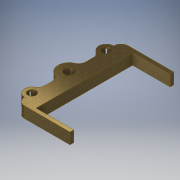
# Autodesk Inventor part: AlteredPlatformATEdit
Saved by Autodesk Inventor 2018 (Build 220112000, 112)
## iProperties
Created: 2017-10-12
Part Number: AlteredPlatformATEdit
Material: Generic
Document SubType Name: Modeling
Designer: 1452927
Density: 1 g/cm^3
Appearance: Foil Gold
Author: 1452927
Autodesk Inventor part; units mm, degrees
ref_plane "YZ Plane" through (0, 0, 0) normal (1, 0, 0) x (0, 1, 0)
sketch "Sketch1" plane through (0, 0, 0) normal (0, 1, 0) x (-1, 0, 0)
  circle A0 centre (0, 0) radius 8.0645
  circle A1 centre (0, -63.5) radius 6.985
  circle A2 centre (0, 63.5) radius 6.985
  line L0 (-39.6048, 88.9) -> (39.6048, 88.9)
  line L1 (39.6048, 88.9) -> (39.6048, -88.9)
  line L2 (39.6048, -88.9) -> (-39.6048, -88.9)
  line L3 (-39.6048, -88.9) -> (-39.6048, 88.9)
  line L4 (-39.6048, 88.9) -> (39.6048, -88.9) construction
  line L5 (39.6048, 88.9) -> (-39.6048, -88.9) construction
  line L6 (10.9754, 63.5) -> (10.9754, 0) construction
  point P0 (0, 0)
  point P1 (0, 0)
  point P2 (0, 63.5)
  dimension "d0" = 16.129
  dimension "d1" = 13.97
  dimension "d2" = 13.97
  dimension "d28" = 177.8
  dimension "d30" = 25.4
  dimension "d31" = 25.4
  constraints: 14 end point, 4 midpoint, 3 centre point, 2 coincident, 2 parallel, 1 horizontal, 1 perpendicular, 1 vertical, 4 other
  measures "d0" diameter of A0
  measures "d1" diameter of A1
  measures "d2" diameter of A2
  measures "d28" distance of L0.end L1.end
  measures "d30" distance from line of L0 point (0, 63.5)
  measures "d31" distance from line of L2 point (0, -63.5)
extrude "Extrusion4" add sketch "Sketch1" along normal blind 19.05
ref_plane "Work Plane2" through (0, 19.05, 0) normal (0, 1, 0) x (1, 0, 0)
sketch "Sketch2" plane through (0, 19.05, 0) normal (0, 1, 0) x (1, 0, 0)
  circle A0 centre (-11.2395, 0) radius 1.25
  circle A1 centre (0, 0) radius 7.94 projected
  circle A2 centre (5.6197, -9.7337) radius 1.25
  circle A3 centre (5.6198, 9.7337) radius 1.25
  dimension "d11" = 2.5
  dimension "d12" = 11.2395
  dimension "d15" = 360
  constraints: 3 centre point, 7 other
  measures "d11" diameter of A0
  measures "d12" distance of A0.centre A1.centre
ref_plane "Work Plane1" through (0, 19.05, 0) normal (0, 1, 0) x (1, 0, 0)
extrude "Extrusion5" cut sketch "Sketch2" against normal up to next contours A0 | A2 | A3
sketch "Sketch6" plane through (0, 19.05, 0) normal (0, 1, 0) x (1, 0, 0)
  line L0 (0, -38.1) -> (0, -18.8395)
  line L1 (0, 18.8395) -> (0, 38.1)
  line L2 (39.6048, 88.9) -> (-39.6048, 88.9) projected
  line L3 (0, 88.9) -> (-39.6048, 88.9)
  line L4 (-39.6048, -88.9) -> (39.6048, -88.9) projected
  line L5 (-39.6048, 88.9) -> (-39.6048, -88.9)
  line L6 (-39.6048, -88.9) -> (0, -88.9)
  circle A0 centre (0, 0) radius 8.0645 projected
  arc A1 (0, 18.8395) -> (0, -18.8395) centre (0, 0) ccw
  arc A2 (0, -50.8) -> (0, -76.2) centre (0, -63.5) ccw
  line L7 (0, -38.1) -> (0, -50.8)
  line L8 (0, -76.2) -> (0, -88.9)
  arc A3 (0, 76.2) -> (0, 50.8) centre (0, 63.5) ccw
  line L9 (0, 88.9) -> (0, 76.2)
  line L10 (0, 50.8) -> (0, 38.1)
  circle A4 centre (0, 63.5) radius 6.477
  circle A5 centre (0, -63.5) radius 6.477
  circle A6 centre (-11.2395, 0) radius 1.25 projected
  point P0 (0, 0)
  dimension "d41" = 25.4
  dimension "d42" = 25.4
  dimension "d44" = 12.954
  dimension "d45" = 12.954
  dimension "d77" = 6.35
  constraints: 18 end point, 6 point on circle, 5 centre point, 4 coincident, 4 point on line, 3 collinear, 3 vertical, 2 midpoint, 1 perpendicular
  measures "d41" diameter of A2
  measures "d42" diameter of A3
  measures "d44" diameter of A4
  measures "d45" diameter of A5
extrude "Extrusion6" cut sketch "Sketch6" against normal blind 19.05 contours L7 A2 L8 L4 L5 L2 L9 A3 L10 L1 A1 L0
fillet "Fillet5" radius 12.7 4 edges at (0, 9.525, 50.8) (0, 9.525, -50.8) (0, 9.525, -18.8395) (0, 9.525, 18.8395)
sketch "Sketch8" plane through (0, 19.05, -88.9) normal (-1, 0, 0) x (0, 0, 1)
  line L0 (33.355, -16.3528) -> (33.355, -2.5052) projected
  line L1 (15.575, -2.511) -> (15.575, -16.351) projected
  line L2 (27.5747, -16.3528) -> (27.5747, -2.5052)
  line L3 (21.1759, -16.351) -> (21.1759, -2.511)
  line L4 (33.355, -16.3528) -> (27.5747, -16.3528)
  line L5 (33.355, -2.5052) -> (27.5747, -2.5052)
  line L6 (15.575, -16.351) -> (21.1759, -16.351)
  line L7 (21.1759, -2.511) -> (15.575, -2.511)
  point P0 (88.9, -19.05)
  constraints: 12 end point, 2 parallel, 1 horizontal, 1 perpendicular
extrude "Extrusion7" cut sketch "Sketch8" along normal up to next
mirror "Mirror1" about plane through (0, 0, 0) normal (0, 0, 1) of "Extrusion7"
fillet "Fillet6" radius 12.7 2 edges at (0, 9.525, 88.9) (0, 9.525, -88.9)
sketch "Sketch12" plane through (0, 19.05, 0) normal (0, 1, 0) x (1, 0, 0)
  line L0 (39.6048, -88.9) -> (39.6048, 88.9) projected
  line L1 (39.6048, -82.55) -> (19.685, -82.55)
  line L2 (19.685, -82.55) -> (19.685, 82.55)
  line L3 (19.685, 82.55) -> (39.6048, 82.55)
  line L4 (39.6048, 82.55) -> (39.6048, -82.55)
  line L5 (39.6048, 88.9) -> (12.7, 88.9) projected
  line L6 (12.7, -88.9) -> (39.6048, -88.9) projected
  circle A0 centre (0, -63.5) radius 6.985 projected
  point P0 (0, 0)
  dimension "d72" = 6.35
  dimension "d73" = 6.35
  dimension "d74" = 12.7
  constraints: 8 end point, 2 parallel, 1 horizontal, 1 perpendicular, 1 point on line
  measures "d72" distance between parallel lines of L5 L3
  measures "d73" distance between parallel lines of L1 L6
  measures "d74" distance edge to line of A0 L2
extrude "Extrusion10" cut sketch "Sketch12" against normal up to next contours L1 L2 L3 L0
sketch "Sketch13" plane through (39.6048, 0, 88.9) normal (1, 0, 0) x (0, 0, -1)
  line L0 (0, 0) -> (0, 19.05) projected
  line L1 (171.45, 0) -> (6.35, 0) projected
  line L2 (0, 19.05) -> (6.35, 19.05)
  line L3 (6.35, 19.05) -> (6.35, 0)
  line L4 (6.35, 0) -> (0, 0)
  line L5 (0, 0) -> (0, 19.05)
  line L6 (171.45, 19.05) -> (171.45, 0) projected
  line L7 (177.8, 19.05) -> (177.8, 0) projected
  line L8 (171.45, 19.05) -> (177.8, 19.05)
  line L9 (177.8, 19.05) -> (177.8, 0)
  line L10 (177.8, 0) -> (171.45, 0)
  line L11 (171.45, 0) -> (171.45, 19.05)
  point P0 (88.9, 0)
  constraints: 16 end point, 4 parallel, 2 horizontal, 2 perpendicular
extrude "Extrusion11" add sketch "Sketch13" along normal blind 50.8
sketch "Sketch14" plane through (19.685, 19.05, 82.55) normal (1, 0, 0) x (0, 0, -1)
  line L0 (0, -19.05) -> (0, 0) projected
  line L1 (0, 0) -> (165.1, 0) projected
  line L2 (165.1, 0) -> (165.1, -19.05) projected
  line L3 (165.1, -19.05) -> (0, -19.05) projected
  point P0 (82.55, -19.05)
extrude "Extrusion12" add sketch "Sketch14" along normal blind 6.35
body "Solid2"
